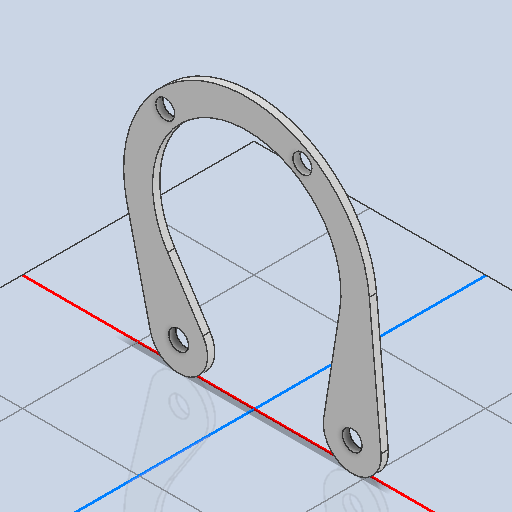
# Autodesk Inventor part: Reservoir Mount
Saved by Autodesk Inventor 2026 (Build 300175000, 175)
## iProperties
Created: 2025-04-08
Part Number: Reservoir Mount
Material: Generic
Document SubType Name: Modeling
Designer: avere
Density: 1 g/cm^3
Appearance: Default
Author: avere
Autodesk Inventor part; units mm, degrees
ref_plane "YZ Plane" through (0, 0, 0) normal (1, 0, 0) x (0, 1, 0)
ref_plane "XZ Plane" through (0, 0, 0) normal (0, 1, 0) x (-1, 0, 0)
ref_plane "XY Plane" through (0, 0, 0) normal (0, 0, 1) x (1, 0, 0)
sketch "main" plane through (0, 0, 0) normal (0, 0, 1) x (1, 0, 0)
  circle A0 centre (-12.7091, -24.4332) radius 2.1844
  circle A1 centre (25.3909, -24.4332) radius 2.1844
  arc A2 (19.133, -23.3552) -> (31.7154, -23.8647) centre (25.3909, -24.4332) ccw
  arc A3 (-18.8897, -25.8904) -> (-7.3754, -20.9874) centre (-12.7091, -24.4332) ccw
  arc A4 (29.1539, 4.6304) -> (-24.0536, -3.989) centre (2.2439, 2.2114) ccw
  line L0 (29.1539, 4.6304) -> (31.7154, -23.8647)
  line L1 (-24.0536, -3.989) -> (-18.8897, -25.8904)
  arc A5 (22.6597, -1.0109) -> (-15.1169, -9.0043) centre (2.2439, 2.2114) ccw
  line L2 (19.133, -23.3552) -> (22.6597, -1.0109)
  line L3 (-7.3754, -20.9874) -> (-15.1169, -9.0043)
  circle A6 centre (-15.6258, 17.9972) radius 2.0955
  circle A7 centre (14.445, 22.6967) radius 2.0955
  point P0 (4.9022, -14.671)
  dimension "d0" = 12.7
  dimension "d1" = 12.7
  dimension "d2" = 6.35
  dimension "d5" = 4.191
  dimension "d6" = 23.8436
  dimension "d7" = 4.191
  dimension "d8" = 23.8436
  measures "d0" diameter of A2
  measures "d1" diameter of A3
  measures "d2" radial gap between concentric circles of A4 A5
  measures "d5" diameter of A6
  measures "d6" distance of A4.centre A6.centre
  measures "d7" diameter of A7
  measures "d8" distance of A4.centre A7.centre
sketch "Sketch1" plane through (0, 0, 0) normal (0, 0, 1) x (1, 0, 0)
  circle A0 centre (-14.953, -26.6446) radius 2.1844
  circle A1 centre (23.147, -26.6446) radius 2.1844
  arc A2 (16.8891, -25.5667) -> (29.4715, -26.0761) centre (23.147, -26.6446) ccw
  arc A3 (-21.1336, -28.1018) -> (-9.6193, -23.1988) centre (-14.953, -26.6446) ccw
  arc A4 (26.9101, 2.4189) -> (-26.2975, -6.2004) centre (0, 0) ccw
  line L0 (26.9101, 2.4189) -> (29.4715, -26.0761)
  line L1 (-26.2975, -6.2004) -> (-21.1336, -28.1018)
  arc A5 (20.4158, -3.2223) -> (-17.3608, -11.2157) centre (0, 0) ccw
  line L2 (16.8891, -25.5667) -> (20.4158, -3.2223)
  line L3 (-9.6193, -23.1988) -> (-17.3608, -11.2157)
  circle A6 centre (-17.8696, 15.7858) radius 2.0955
  circle A7 centre (12.2011, 20.4853) radius 2.0955
  constraints: 1 other
extrude "Extrusion1" add sketch "Sketch1" along normal blind 1.5875
body "Solid1"
